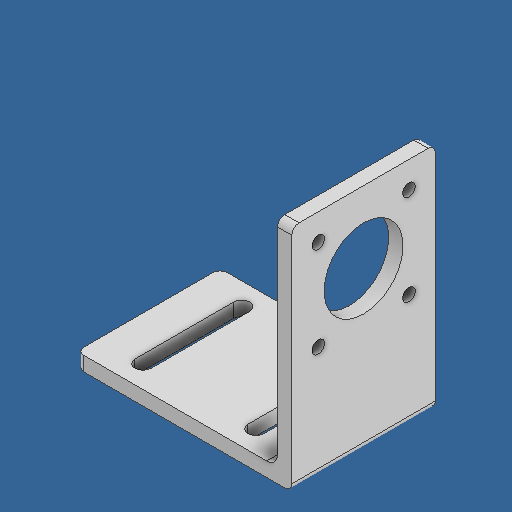
# Autodesk Inventor part: BRACKET__MOTOR
Saved by Autodesk Inventor 2025 (Build 290162000, 162)
## iProperties
Created: 2026-01-21
Part Number: BRACKET__MOTOR
Material: Genérico
Document SubType Name: Modeling
Designer: HP
Density: 1 g/cm^3
Appearance: Valor por defecto
Author: HP
Autodesk Inventor part; units mm, degrees
ref_plane "YZ Plane" through (0, 0, 0) normal (1, 0, 0) x (0, 1, 0)
ref_plane "XZ Plane" through (0, 0, 0) normal (0, 1, 0) x (-1, 0, 0)
ref_plane "XY Plane" through (0, 0, 0) normal (0, 0, 1) x (1, 0, 0)
sketch "Boceto1" plane through (0, 0, 0) normal (1, 0, 0) x (0, 1, 0)
  line L0 (-6.321, 6.321) -> (6.321, 6.321) construction
  line L1 (6.321, 6.321) -> (6.321, -6.321) construction
  line L2 (6.321, -6.321) -> (-6.321, -6.321) construction
  line L3 (-6.321, -6.321) -> (-6.321, 6.321) construction
  line L4 (-6.321, 6.321) -> (6.321, -6.321) construction
  line L5 (6.321, 6.321) -> (-6.321, -6.321) construction
  circle A0 centre (6.321, -6.321) radius 0.875
  line L6 (0, 0) -> (7.9878, 0) construction
  circle A1 centre (6.321, 6.321) radius 0.875
  line L7 (0, 0) -> (0, -13.4562) construction
  circle A2 centre (-6.321, -6.321) radius 0.875
  circle A3 centre (-6.321, 6.321) radius 0.875
  circle A4 centre (0, 0) radius 5.5
  line L8 (10, 10) -> (-20, 10)
  line L9 (-20, 10) -> (-20, -10)
  line L10 (-20, -10) -> (10, -10)
  line L11 (10, -10) -> (10, 10)
  dimension "d0" = 12.642
  dimension "d1" = 12.642
  dimension "d2" = 1.75
  dimension "d3" = 11
  dimension "d4" = 30
  dimension "d5" = 20
  dimension "d6" = 10
  dimension "d7" = 10
  constraints: 24 end point, 5 centre point, 4 parallel, 3 coincident, 3 horizontal, 3 symmetric about line, 2 midpoint, 2 perpendicular, 1 vertical, 3 other
  measures "d0" distance of L1.end L2.end
  measures "d1" distance of L0.end L1.end
  measures "d2" diameter of A0
  measures "d3" diameter of A4
  measures "d4" distance of L10.end L9.end
  measures "d5" distance of L9.end L8.end
  measures "d6" distance from line of L6.start L8
  measures "d7" distance from line of L6.start L11
extrude "Extrusión1" add sketch "Boceto1" along normal blind 2
sketch "Boceto2" plane through (0, -20, -10) normal (0, -1, 0) x (1, 0, 0)
  line L0 (2, 0) -> (2, 20) projected
  line L1 (2, 20) -> (-28, 20)
  line L2 (-28, 20) -> (-28, 0)
  line L3 (-28, 0) -> (2, 0)
  line L4 (2, 0) -> (2, 20)
  point P0 (0, 10)
  dimension "d10" = 30
  dimension "d11" = 20
  constraints: 8 end point, 2 parallel, 1 horizontal, 1 perpendicular
  measures "d10" distance of L3.end L2.end
  measures "d11" distance of L2.end L1.end
extrude "Extrusión2" add sketch "Boceto2" along normal blind 2
sketch "Boceto3" plane through (0, -20, -10) normal (0, 1, 0) x (1, 0, 0)
  line L0 (0, -20) -> (0, 0) projected
  line L1 (-28, 0) -> (0, 0) projected
  line L2 (-28, -20) -> (-28, 0) projected
  line L3 (0, -20) -> (-28, -20) projected
  line L4 (-6.125, -3.125) -> (-6.125, -16.875) construction
  line L5 (-7.25, -3.125) -> (-7.25, -16.875)
  line L6 (-5, -16.875) -> (-5, -3.125)
  arc A0 (-5, -3.125) -> (-7.25, -3.125) centre (-6.125, -3.125) ccw
  arc A1 (-7.25, -16.875) -> (-5, -16.875) centre (-6.125, -16.875) ccw
  line L7 (-21.875, -3.125) -> (-21.875, -16.875) construction
  line L8 (-23, -3.125) -> (-23, -16.875)
  line L9 (-20.75, -16.875) -> (-20.75, -3.125)
  arc A2 (-20.75, -3.125) -> (-23, -3.125) centre (-21.875, -3.125) ccw
  arc A3 (-23, -16.875) -> (-20.75, -16.875) centre (-21.875, -16.875) ccw
  point P0 (0, -10)
  point P1 (-6.125, -10)
  point P2 (-21.875, -10)
  point P3 (-21.875, -18)
  point P4 (-21.875, -2)
  point P5 (-6.125, -18)
  point P6 (-6.125, -2)
  dimension "d14" = 2.25
  dimension "d15" = 2.25
  dimension "d16" = 5
  dimension "d17" = 2
  dimension "d18" = 2
  dimension "d19" = 2
  dimension "d20" = 2
  dimension "d21" = 5
  constraints: 16 end point, 12 point on circle, 8 tangent, 4 centre point, 3 parallel, 2 midpoint, 1 vertical
  measures "d14" diameter of A1
  measures "d15" diameter of A3
  measures "d16" distance between parallel lines of L8 L2
  measures "d17" distance from line of L3 point (-21.875, -18)
  measures "d18" distance from line of L1 point (-21.875, -2)
  measures "d19" distance from line of L3 point (-6.125, -18)
  measures "d20" distance from line of L1 point (-6.125, -2)
  measures "d21" distance between parallel lines of L6 L0
extrude "Extrusión3" cut sketch "Boceto3" against normal through all contours A0 L6 A1 L5 | A2 L9 A3 L8
fillet "Empalme1" radius 1.5 1 edges at (0, -20, 0)
fillet "Empalme2" radius 1 5 edges at (1, 10, 10) (1, 10, -10) (-28, -21, 10) (-28, -21, -10) (2, -22, 0)
